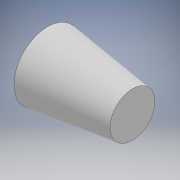
# Autodesk Inventor part: cup
Saved by Autodesk Inventor 2018 (Build 220112000, 112)
## iProperties
Created: 2017-11-15
Part Number: cup
Material: Generic
Document SubType Name: Modeling
Designer: Prakash
Density: 1 g/cm^3
Appearance: Default
Author: Prakash
Autodesk Inventor part; units mm, degrees
ref_plane "YZ Plane" through (0, 0, 0) normal (1, 0, 0) x (0, 1, 0)
ref_plane "XZ Plane" through (0, 0, 0) normal (0, 1, 0) x (-1, 0, 0)
ref_plane "XY Plane" through (0, 0, 0) normal (0, 0, 1) x (1, 0, 0)
sketch "Sketch1" plane through (0, 0, 0) normal (0, 1, 0) x (-1, 0, 0)
  line L0 (0, 0) -> (0, -63.5)
  line L1 (120.65, 15.875) -> (120.65, -79.375)
  line L2 (0, -63.5) -> (120.65, -79.375)
  line L3 (0, 0) -> (120.65, 15.875)
  line L4 (120.65, -31.75) -> (0, -31.75)
  line L5 (0, -31.75) -> (9.25, -31.75)
  line L6 (120.65, -31.75) -> (28.15, -31.75)
  line L7 (28.15, 3.7039) -> (28.15, -67.2039)
  line L8 (19.15, 9.75) -> (19.15, -73.25)
  line L9 (19.15, -73.25) -> (37.15, -73.25)
  line L10 (37.15, -73.25) -> (37.15, 9.75)
  line L11 (37.15, 9.75) -> (19.15, 9.75)
  line L12 (19.15, 9.75) -> (37.15, -73.25) construction
  line L13 (19.15, -73.25) -> (37.15, 9.75) construction
  dimension "d0" = 63.5
  dimension "d1" = 95.25
  dimension "d2" = 120.65
  dimension "d6" = 92.5
  dimension "d7" = 70.9079
  dimension "d8" = 83
  dimension "d9" = 18
  constraints: 28 end point, 4 midpoint, 4 point on line, 4 vertical, 2 parallel, 1 equal length, 1 perpendicular
  measures "d0" distance of L0.start L0.end
  measures "d1" distance of L1.start L1.end
  measures "d2" distance between parallel lines of L0 L1
  measures "d6" distance of L4.start L6.end
  measures "d7" distance of L7.start L7.end
  measures "d8" distance of L8.start L8.end
  measures "d9" distance of L9.end L8.end
revolve "Revolution1" add sketch "Sketch1" angle 360 about axis through (-120.65, 0, -31.75) along (1, 0, 0) contours L3 L8 L4 L0 | L4 L8 L2 L0 | L3 L7 L4 L8 | L3 L10 L4 L7 | L4 L7 L2 L8 | L3 L1 L4 L10 | L4 L10 L2 L7 | L4 L1 L2 L10
body "Solid1"
